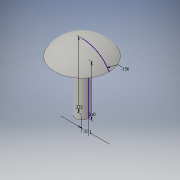
# Autodesk Inventor part: Linkage Peg
Saved by Autodesk Inventor 2016 (Build 200138000, 138)
## iProperties
Created: 2018-01-09
Part Number: Linkage Peg
Material: Generic
Document SubType Name: Modeling
Designer: sun01147
Density: 1 g/cm^3
Appearance: Default
Mass: 0.0505621 g
Surface Area: 1.15245 cm^2
Volume: 0.0505621 cm^3
Author: sun01147
Autodesk Inventor part; units mm, degrees
ref_plane "YZ Plane" through (0, 0, 0) normal (1, 0, 0) x (0, 1, 0)
ref_plane "XZ Plane" through (0, 0, 0) normal (0, 1, 0) x (-1, 0, 0)
ref_plane "XY Plane" through (0, 0, 0) normal (0, 0, 1) x (1, 0, 0)
sketch "Sketch1" plane through (0, 0, 0) normal (0, 0, 1) x (1, 0, 0)
  line L0 (0, 0) -> (0.7937, 0)
  line L1 (0.7937, 0) -> (0.7937, 6.35)
  line L2 (0, 0) -> (0, 8.255)
  line L3 (0.7937, 6.35) -> (3.3893, 6.35)
  arc A0 (3.3893, 6.35) -> (0, 8.255) centre (0, 4.2875) ccw
  dimension "d0" = 0.7937
  dimension "d1" = 6.35
  dimension "d2" = 8.255
  dimension "d3" = 3.9675
  constraints: 8 end point, 2 horizontal, 2 point on circle, 2 vertical, 1 centre point, 1 line through centre
  measures "d0" distance of L0.start L0.end
  measures "d1" distance of L0.end L1.end
  measures "d2" distance of L0.start L2.end
  measures "d3" radius of A0
revolve "Revolution1" add sketch "Sketch1" angle 360 about axis through (0, 0, 0) along (0, 1, 0)
body "Solid1"
